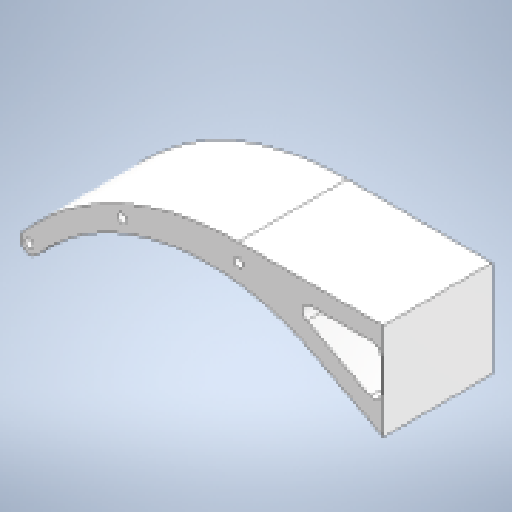
# Autodesk Inventor part: tesaki_sukima
Saved by Autodesk Inventor 2025.1 (Build 291241000, 241)
## iProperties
Created: 2024-09-04
Part Number: tesaki_sukima
Material: ABS プラスチック
Document SubType Name: Modeling
Designer: right
Density: 1.06 g/cm^3
Appearance: 滑らか - 白
Author: right
Autodesk Inventor part; units mm, degrees
ref_plane "YZ Plane" through (0, 0, 0) normal (1, 0, 0) x (0, 1, 0)
ref_plane "XZ Plane" through (0, 0, 0) normal (0, 1, 0) x (-1, 0, 0)
ref_plane "XY Plane" through (0, 0, 0) normal (0, 0, 1) x (1, 0, 0)
sketch "スケッチ1" plane through (0, 0, 0) normal (0, 0, 1) x (1, 0, 0)
  circle A0 centre (-57.5501, -12.4578) radius 1.1 projected
  circle A1 centre (-3.4499, 10.3504) radius 1.1 projected
  circle A2 centre (-33.4499, 5.2266) radius 1.1 projected
  line L0 (15.1751, 9.9578) -> (31.5501, 9.9578) projected
  arc A3 (33.5501, 7.9578) -> (31.5501, 9.9578) centre (31.5501, 7.9578) ccw projected
  line L1 (33.5501, 7.9578) -> (33.5501, -0.7755) projected
  arc A4 (30.6089, -2.5402) -> (33.5501, -0.7755) centre (31.5501, -0.7755) ccw projected
  line L2 (30.6089, -2.5402) -> (14.2339, 6.1931) projected
  arc A5 (15.1751, 9.9578) -> (14.2339, 6.1931) centre (15.1751, 7.9578) ccw projected
  line L3 (57.5501, 14.9578) -> (-3.4499, 14.9578) projected
  arc A6 (-3.4499, 14.9578) -> (-59.4499, -10.8327) centre (-3.4499, -58.735) ccw projected
  arc A7 (-59.4499, -10.8327) -> (-55.6581, -14.0919) centre (-57.5501, -12.4578) ccw projected
  arc A8 (16.4506, -0.6558) -> (-55.6581, -14.0919) centre (-11.1964, -52.494) ccw projected
  line L4 (16.4506, -0.6558) -> (35.3736, -10.7481) projected
  arc A9 (35.3736, -10.7481) -> (39.0501, -8.5422) centre (36.5501, -8.5422) ccw projected
  line L5 (39.0501, -8.5422) -> (39.0501, 7.9578) projected
  arc A10 (41.0501, 9.9578) -> (39.0501, 7.9578) centre (41.0501, 7.9578) ccw projected
  line L6 (41.0501, 9.9578) -> (57.5501, 9.9578) projected
  arc A11 (57.5501, 9.9578) -> (57.5501, 14.9578) centre (57.5501, 12.4578) ccw projected
  circle A12 centre (36.5501, -8.5422) radius 1.1 projected
  circle A13 centre (57.5501, 12.4578) radius 1.1 projected
  circle A14 centre (36.5501, 12.4578) radius 1.1 projected
  line L7 (34.0501, -10.0422) -> (34.0501, 14.9578)
  line L8 (34.0501, 12.4578) -> (34.0501, -8.5422) projected
  circle A15 centre (-57.5501, -12.4578) radius 0.8
  circle A16 centre (-33.4499, 5.2266) radius 0.8
  circle A17 centre (-3.4499, 10.3504) radius 0.8
  circle A18 centre (30.6089, 12.4578) radius 1.1 projected
  circle A19 centre (30.6089, -5.3736) radius 1.1 projected
  circle A20 centre (6.5501, 10.3504) radius 1.1 projected
  circle A21 centre (30.6089, 12.4578) radius 0.8
  circle A22 centre (6.5501, 10.3504) radius 0.8
  circle A23 centre (30.6089, -5.3736) radius 0.8
  point P0 (0, 0)
  dimension "d0" = 1.6
  dimension "d1" = 1.6
  dimension "d2" = 1.6
  dimension "d5" = 1.6
  dimension "d6" = 1.6
  dimension "d7" = 1.6
  constraints: 6 centre point, 6 coincident, 3 point on line, 2 end point, 1 vertical
  measures "d0" diameter of A15
  measures "d1" diameter of A16
  measures "d2" diameter of A17
  measures "d5" diameter of A21
  measures "d6" diameter of A22
  measures "d7" diameter of A23
ref_plane "作業平面1" through (-60.0501, -14.9578, 28.2) normal (0, 0, 1) x (1, 0, 0)
extrude "押し出し1" add sketch "スケッチ1" along normal up to surface (28.2 mm away) contours A0 | A1 | A2 | L7 L4 A8 A7 A6 L3 | A18 | A19 | A20
fillet "フィレット1" radius 2.5 2 edges at (34.0501, 14.9578, 14.1) (34.0501, -10.0422, 14.1)
